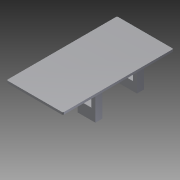
# Autodesk Inventor part: M201101-terminals
Saved by Autodesk Inventor 2014 (Build 180170000, 170)
## iProperties
Category: PARTsolutions
Company: NKKSWITCHES
Created: 2013-12-29
Part Number: M201101-terminals
Catalog Web Link: www.cadenas.de
Description: Bushing Mount Miniature Toggles-Terminals-Series M - Miniature Toggles
Vendor: NKKSWITCHES
Document SubType Name: Modeling
Designer: PARTuser1
Manufacturer: NKKSWITCHES
Density: 1 g/cm^3
Material: Generic
Appearance: RGB(192.00000375509219,192.00000375509219,192.00000375509219)
PSOL_IDENT_0: {$CADENAS_DATA\23d-libs\nkkswitches\toggle\m\parts\m_bt_terminal.prj},227 {VTYP=3D},{NB=M201101-term
PSOL_IDENT_1: inals},{LINA=M201101-terminals},{NN=Bushing Mount Miniature Toggles-Terminals},{DATE=28.05.2013 12:0
PSOL_IDENT_2: 6:56},{GEOMDATE=28.05.2013 12:06:56},{VERSION=},{LINEID=10},{LINESUBID=-1},{WBVAR=PLS,CRCTS,TRMNLS}
PSOL_IDENT_3: {NB=M201101-terminals},{LINA=M201101-terminals},{KT=DUMMY},{PN=M201101},{SRS=M20},{PLS=1},{CRCTSALG
PSOL_IDENT_4: ='1','1 - ON/NONE/OFF','2','2 - ON/NONE/ON','3','3 - ON/OFF/ON','5','5 - ON/NONE/(ON)','8','8 - (ON)
PSOL_IDENT_5: /OFF/(ON)','9','9 - ON/OFF/(ON)','4', '4 - ON/ON/ON','6','6 - (ON)/ON/(ON)','7','7 - ON/ON/(ON)'},{C
PSOL_IDENT_6: RCTS=1},{TRMNLSALG='01','01 - Solder Lug','02','02 - Quick Connect','03','03 - .250\" (6.35mm) Strai
PSOL_IDENT_7: ght PC','05', '05 - .425\" (10.8mm) Wirewrap','06', '06 - .750\" (19.05mm) Wirewrap','07', '07 - .96
PSOL_IDENT_8: 4\" (24.5mm) Wirewrap','08', '08 - 1.062\" (27.0mm) Wirewrap'},{TRMNLS=01},{WIDTH=0.512},{HEIGHT=0.3
PSOL_IDENT_9: 7},{LENGTH=0.311},{A=0},{TRMNLNOH=1},{POS=0},{TRMNLOV=2}
CNS_NN: Bushing Mount Miniature Toggles-Terminals
CNS_NT: Series M - Miniature Toggles
CNS_NB: M201101-terminals
CNS_NBSYN: $PN.-terminals
CNS_LINA: M201101-terminals
CNS_PN: M201101
CNS_SRS: M20
CNS_PLS: 1 - SPST/SPDT
CNS_CRCTSALG: '1','1 - ON/NONE/OFF','2','2 - ON/NONE/ON','3','3 - ON/OFF/ON','5','5 - ON/NONE/(ON)','8','8 - (ON)/OFF/(ON)','9','9 - ON/OFF/(ON)','4', '4 - ON/ON/ON','6','6 - (ON)/ON/(ON)','7','7 - ON/ON/(ON)'
CNS_CRCTS: 1 - ON/NONE/OFF
CNS_TRMNLSALG: '01','01 - Solder Lug','02','02 - Quick Connect','03','03 - .250" (6.35mm) Straight PC','05', '05 - .425" (10.8mm) Wirewrap','06', '06 - .750" (19.05mm) Wirewrap','07', '07 - .964" (24.5mm) Wirewrap','08', '08 - 1.062" (27.0mm) Wirewrap'
CNS_TRMNLS: 01 - Solder Lug
CNS_WIDTH: 0.512
CNS_HEIGHT: 0.370
CNS_LENGTH: 0.311
CNS_A: 0.000
CNS_TRMNLNOH: 1.000
CNS_POS: 0.000
CNS_TRMNLOV: 2.000
SUPPLIER: NKKSWITCHES
ARTICLENO: M201101-terminals
BOMINFO: M201101-terminals
CREATOR: CADENAS GmbH
Title: M201101-terminals
Author: Cadenas PARTsolutions
Comments: Series M - Miniature Toggles
Autodesk Inventor part; units mm, degrees
sketch "Sketch_2" plane through (0, 0, 0) normal (0, 1, 0) x (-1, 0, 0)
  line L0 (3.1877, -6.1184) -> (3.1877, 6.1184)
  arc A0 (3.1877, 6.1184) -> (3.0577, 6.2484) centre (3.0577, 6.1184) ccw
  line L1 (3.0577, 6.2484) -> (-3.0577, 6.2484)
  arc A1 (-3.0577, 6.2484) -> (-3.1877, 6.1184) centre (-3.0577, 6.1184) ccw
  line L2 (-3.1877, 6.1184) -> (-3.1877, -6.1184)
  arc A2 (-3.1877, -6.1184) -> (-3.0577, -6.2484) centre (-3.0577, -6.1184) ccw
  line L3 (-3.0577, -6.2484) -> (3.0577, -6.2484)
  arc A3 (3.0577, -6.2484) -> (3.1877, -6.1184) centre (3.0577, -6.1184) ccw
  constraints: 8 end point, 8 point on circle, 4 centre point
extrude "Extrusion1" add sketch "Sketch_2" along normal blind 0.254
sketch "Sketch_12" plane through (0, 0, -4.699) normal (0, 0, 1) x (1, 0, 0)
  line L0 (-1.0033, 0) -> (-1.0033, -4.2418)
  line L1 (-1.0033, -4.2418) -> (1.0033, -4.2418)
  line L2 (1.0033, -4.2418) -> (1.0033, 0)
  line L3 (1.0033, 0) -> (-1.0033, 0)
  line L4 (-0.5461, -1.2446) -> (-0.5461, -3.2512)
  line L5 (-0.5461, -3.2512) -> (0.5461, -3.2512)
  line L6 (0.5461, -3.2512) -> (0.5461, -1.2446)
  line L7 (0.5461, -1.2446) -> (-0.5461, -1.2446)
  constraints: 16 end point
extrude "Extrusion2" add sketch "Sketch_12" along normal mid plane 0.7874
sketch "Sketch_14" plane through (0, 0, 0) normal (0, 0, 1) x (1, 0, 0)
  line L0 (-1.0033, 0) -> (-1.0033, -4.7498)
  line L1 (-1.0033, -4.7498) -> (1.0033, -4.7498)
  line L2 (1.0033, -4.7498) -> (1.0033, 0)
  line L3 (1.0033, 0) -> (-1.0033, 0)
  line L4 (-0.5461, -1.4986) -> (-0.5461, -3.5052)
  line L5 (-0.5461, -3.5052) -> (0.5461, -3.5052)
  line L6 (0.5461, -3.5052) -> (0.5461, -1.4986)
  line L7 (0.5461, -1.4986) -> (-0.5461, -1.4986)
  constraints: 16 end point
extrude "Extrusion3" add sketch "Sketch_14" along normal mid plane 0.7874
ref_plane "to_base_XY" through (0, 0, 0) normal (0, 1, 0) x (1, 0, 0)
ref_plane "to_base_YZ" through (0, 0, 0) normal (1, 0, 0) x (0, 0, -1)
ref_plane "to_base_ZX" through (0, 0, 0) normal (0, 0, -1) x (0, 1, 0)
body "Solid1"
